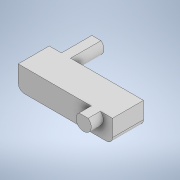
# Autodesk Inventor part: rpi_base_front_gambi
Saved by Autodesk Inventor 2022.1 (Build 261234000, 234)
## iProperties
Created: 2021-07-18
Part Number: rpi_base_front_gambi
Material: Generic
Document SubType Name: Modeling
Designer: dwbertol
Density: 1 g/cm^3
Appearance: Default
Author: dwbertol
## iProperties of the stored document rpi_base_front_3DPrint.ipt
Created: 2021-07-18
Part Number: rpi_base_front_3DPrint
Material: Generic
Document SubType Name: Modeling
Designer: dwbertol
Density: 1 g/cm^3
Appearance: Default
Author: dwbertol
Autodesk Inventor part; units mm, degrees
ref_plane "YZ Plane" through (0, 0, 0) normal (1, 0, 0) x (0, 1, 0)
ref_plane "XZ Plane" through (0, 0, 0) normal (0, 1, 0) x (-1, 0, 0)
ref_plane "XY Plane" through (0, 0, 0) normal (0, 0, 1) x (1, 0, 0)
sketch "Sketch1" plane through (0, 0, 0) normal (0, 0, 1) x (1, 0, 0)
  circle A0 centre (0, 0) radius 1.25
  circle A1 centre (0, 0) radius 2.75
  line L0 (-1.75, 2.75) -> (1.75, 2.75)
  line L1 (2.75, 1.75) -> (2.75, -1.75)
  line L2 (1.75, -2.75) -> (-1.75, -2.75)
  line L3 (-2.75, -1.75) -> (-2.75, 1.75)
  arc A2 (-1.75, 2.75) -> (-2.75, 1.75) centre (-1.75, 1.75) ccw
  arc A3 (2.75, 1.75) -> (1.75, 2.75) centre (1.75, 1.75) ccw
  arc A4 (1.75, -2.75) -> (2.75, -1.75) centre (1.75, -1.75) ccw
  arc A5 (-2.75, -1.75) -> (-1.75, -2.75) centre (-1.75, -1.75) ccw
  line L4 (-2.75, 1) -> (2.75, 1)
  line L5 (0, 2.75) -> (-11.75, 2.75)
  line L6 (-12.75, 1.75) -> (-12.75, -1.75)
  line L7 (-11.75, -2.75) -> (0, -2.75)
  line L8 (0, -2.75) -> (0, 2.75)
  circle A6 centre (-10, 0) radius 2.75
  circle A7 centre (-10, 0) radius 1.25
  line L9 (-2.75, 1) -> (-12.75, 1)
  arc A8 (-11.75, 2.75) -> (-12.75, 1.75) centre (-11.75, 1.75) ccw
  arc A9 (-12.75, -1.75) -> (-11.75, -2.75) centre (-11.75, -1.75) ccw
  point P0 (-2.75, 0)
  point P1 (0, -2.75)
  point P2 (0.75, 1)
  point P3 (-0.75, 1)
  point P4 (0, 0)
  point P5 (-9.25, 1)
  point P6 (-10.75, 1)
  dimension "d0" = 2.5
  dimension "d1" = 5.5
  dimension "d2" = 1
  dimension "d3" = 1
  dimension "d4" = 1
  dimension "d11" = 1
  dimension "d12" = 2.5
  dimension "d13" = 10
  dimension "d14" = 1
  constraints: 20 end point, 19 tangent, 12 point on circle, 10 centre point, 4 parallel, 4 point on line, 3 coincident, 3 perpendicular, 2 equal radius, 2 horizontal, 2 midpoint, 1 collinear
  measures "d0" diameter of A0
  measures "d1" diameter of A1
  measures "d2" radius of A2
  measures "d3" radius of A3
  measures "d4" radius of A5
  measures "d11" distance from line of L4 point (0, 0)
  measures "d12" diameter of A7
  measures "d13" distance of point (0, 0) A6.centre
  measures "d14" radius of A8
extrude "Extrusion1" add sketch "Sketch1" along normal blind 7.1 contours A0 L8 L4 | A0 L4 L8 picked at (0.0927, -0.4896) picked at (-0.103, -0.4871)
extrude "Extrusion2" add sketch "Sketch1" along normal blind 5.1 contours A0 L8 L4 | A0 L4 A1 L8 | L8 A1 L4 A0 | A0 L4 L8 | L4 L1 A1 | L2 A5 L3 A1 | A1 L1 A4 L2 | A1 L3 L4 | L3 A5 L7 A6 L9 | L7 A9 L6 A6 | A6 L9 A7 | L6 L9 A6 | A7 L9 picked at (0.0927, -0.4896) picked at (2.2166, -0.2967) picked at (-0.204, -2.227) picked at (-0.103, -0.4871) picked at (-7.773, -0.204) picked at (-10.4044, -0.1231)
extrude "Extrusion3" add sketch "Sketch1" against normal blind 5 contours A7 L9 picked at (-10.4044, -0.1231)
equation "\"d12\" = d0"
body "Solid1"
